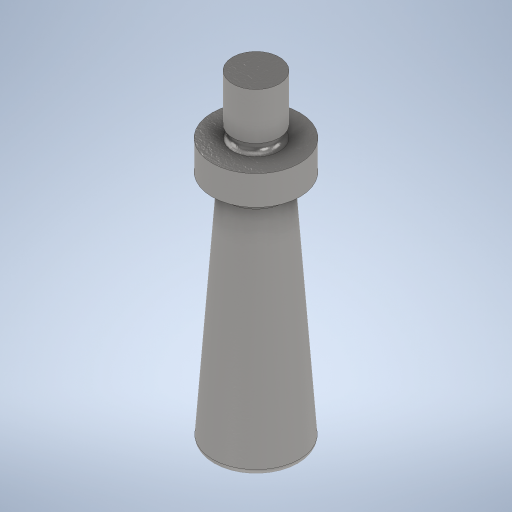
# Autodesk Inventor part: Griff
Saved by Autodesk Inventor 2024 (Build 280153000, 153)
## iProperties
Created: 2024-03-01
Part Number: Griff
Material: Stahl, galvanisiert
Document SubType Name: Modeling
Designer: ffogue
Density: 7.85 g/cm^3
Appearance: Galvanisiert
Author: ffogue
Autodesk Inventor part; units mm, degrees
ref_plane "YZ Plane" through (0, 0, 0) normal (1, 0, 0) x (0, 1, 0)
ref_plane "XZ Plane" through (0, 0, 0) normal (0, 1, 0) x (-1, 0, 0)
ref_plane "XY Plane" through (0, 0, 0) normal (0, 0, 1) x (1, 0, 0)
sketch "Skizze1" plane through (0, 0, 0) normal (0, 1, 0) x (-1, 0, 0)
  line L0 (0, 0) -> (0, -55)
  line L1 (0, 0) -> (4, 0)
  line L2 (4, 0) -> (4, -8)
  arc A0 (4, -8) -> (4, -10) centre (4, -9) ccw
  line L3 (4, -10) -> (7.5, -10)
  line L4 (7.5, -10) -> (7.5, -15)
  line L5 (7.5, -15) -> (4.7029, -15)
  line L6 (4.7029, -15) -> (7.5, -55)
  line L7 (7.5, -55) -> (0, -55)
  point P0 (2, 0)
  dimension "d0" = 4
  dimension "d1" = 5
  dimension "d2" = 8
  dimension "d3" = 15
  dimension "d4" = 8
  dimension "d5" = 10
  dimension "d6" = 55
  dimension "d7" = 15
  constraints: 16 end point, 4 perpendicular, 2 point on circle, 2 point on line, 1 centre point, 1 coincident, 1 horizontal, 1 midpoint, 1 parallel, 1 tangent, 1 vertical
  measures "d0" angle of L6 L0
  measures "d1" distance between parallel lines of L5 L3
  measures "d2" diameter of L2 L0
  measures "d3" diameter of L4 L0
  measures "d4" distance from line of L2.end L1
  measures "d5" distance between parallel lines of L3 L1
  measures "d6" distance from line of L7 point (2, 0)
  measures "d7" diameter of L6.end L0
revolve "Umdrehung1" add sketch "Skizze1" angle 360 about axis through (0, 0, 0) along (0, 0, -1)
fillet "Rundung1" radius 2 1 edges at (4.7029, 0, -15)
fillet "Rundung2" radius 1 1 edges at (7.5, 0, -55)
